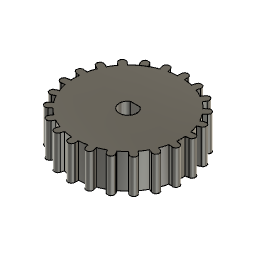
ZahnradProfilVorlage v5 (Autodesk Fusion 360 design; units mm, degrees)
Autodesk Fusion 360 part; units mm, degrees
note: some values were not read from the file. Chosen so that the rebuilt part matches the saved one: which face or edge a step refers to. Set by a fixed rule: which sketch regions a step uses.
sketch "Skizze1" plane through (0, 0, 0) normal (0, 0, 1) x (1, 0, 0)
  circle A0 centre (0, 0) radius 15.5076
  circle A1 centre (0, 16.5076) radius 1
  line L0 (-1, 16.5076) -> (1, 16.5076)
  line L1 (1, 16.5076) -> (1, 15.4753)
  line L2 (1, 15.4753) -> (-1, 15.4753)
  line L3 (-1, 15.4753) -> (-1, 16.5076)
  circle A2 centre (0, 0) radius 2.55
  line L4 (-1.4429, 2.1025) -> (1.4502, 2.0975)
  circle A3 centre (0, 0) radius 17.5076
  line L5 (-3.6912, 16.1206) -> (-3.4004, 15.1302)
  line L6 (-3.4004, 15.1302) -> (-5.3194, 14.5667)
  line L7 (-5.6102, 15.5572) -> (-3.6912, 16.1206)
  circle A4 centre (-4.6507, 15.8389) radius 1
  line L8 (-5.3194, 14.5667) -> (-5.6102, 15.5572)
  line L9 (-8.0834, 14.4277) -> (-7.5253, 13.5593)
  line L10 (-7.5253, 13.5593) -> (-9.2078, 12.478)
  line L11 (-9.7659, 13.3464) -> (-8.0834, 14.4277)
  circle A5 centre (-8.9247, 13.887) radius 1
  line L12 (-9.2078, 12.478) -> (-9.7659, 13.3464)
  line L13 (-11.8207, 11.5659) -> (-11.0406, 10.8899)
  line L14 (-11.0406, 10.8899) -> (-12.3503, 9.3784)
  line L15 (-13.1304, 10.0544) -> (-11.8207, 11.5659)
  circle A6 centre (-12.4756, 10.8102) radius 1
  line L16 (-12.3503, 9.3784) -> (-13.1304, 10.0544)
  line L17 (-14.6004, 7.7671) -> (-13.6614, 7.3383)
  line L18 (-13.6614, 7.3383) -> (-14.4922, 5.519)
  line L19 (-15.4312, 5.9479) -> (-14.6004, 7.7671)
  circle A7 centre (-15.0158, 6.8575) radius 1
  line L20 (-14.4922, 5.519) -> (-15.4312, 5.9479)
  line L21 (-16.1972, 3.3391) -> (-15.1755, 3.1922)
  line L22 (-15.1755, 3.1922) -> (-15.4601, 1.2125)
  line L23 (-16.4819, 1.3594) -> (-16.1972, 3.3391)
  circle A8 centre (-16.3395, 2.3493) radius 1
  line L24 (-15.4601, 1.2125) -> (-16.4819, 1.3594)
  line L25 (-16.4819, -1.3594) -> (-15.4601, -1.2125)
  line L26 (-15.4601, -1.2125) -> (-15.1755, -3.1922)
  line L27 (-16.1972, -3.3391) -> (-16.4819, -1.3594)
  circle A9 centre (-16.3395, -2.3493) radius 1
  line L28 (-15.1755, -3.1922) -> (-16.1972, -3.3391)
  line L29 (-15.4312, -5.9479) -> (-14.4922, -5.519)
  line L30 (-14.4922, -5.519) -> (-13.6614, -7.3383)
  line L31 (-14.6004, -7.7671) -> (-15.4312, -5.9479)
  circle A10 centre (-15.0158, -6.8575) radius 1
  line L32 (-13.6614, -7.3383) -> (-14.6004, -7.7671)
  line L33 (-13.1304, -10.0544) -> (-12.3503, -9.3784)
  line L34 (-12.3503, -9.3784) -> (-11.0406, -10.8899)
  line L35 (-11.8207, -11.5659) -> (-13.1304, -10.0544)
  circle A11 centre (-12.4756, -10.8102) radius 1
  line L36 (-11.0406, -10.8899) -> (-11.8207, -11.5659)
  line L37 (-9.7659, -13.3464) -> (-9.2078, -12.478)
  line L38 (-9.2078, -12.478) -> (-7.5253, -13.5593)
  line L39 (-8.0834, -14.4277) -> (-9.7659, -13.3464)
  circle A12 centre (-8.9247, -13.887) radius 1
  line L40 (-7.5253, -13.5593) -> (-8.0834, -14.4277)
  line L41 (-5.6102, -15.5572) -> (-5.3194, -14.5667)
  line L42 (-5.3194, -14.5667) -> (-3.4004, -15.1302)
  line L43 (-3.6912, -16.1206) -> (-5.6102, -15.5572)
  circle A13 centre (-4.6507, -15.8389) radius 1
  line L44 (-3.4004, -15.1302) -> (-3.6912, -16.1206)
  line L45 (-1, -16.5076) -> (-1, -15.4753)
  line L46 (-1, -15.4753) -> (1, -15.4753)
  line L47 (1, -16.5076) -> (-1, -16.5076)
  circle A14 centre (0, -16.5076) radius 1
  line L48 (1, -15.4753) -> (1, -16.5076)
  line L49 (3.6912, -16.1206) -> (3.4004, -15.1302)
  line L50 (3.4004, -15.1302) -> (5.3194, -14.5667)
  line L51 (5.6102, -15.5572) -> (3.6912, -16.1206)
  circle A15 centre (4.6507, -15.8389) radius 1
  line L52 (5.3194, -14.5667) -> (5.6102, -15.5572)
  line L53 (8.0834, -14.4277) -> (7.5253, -13.5593)
  line L54 (7.5253, -13.5593) -> (9.2078, -12.478)
  line L55 (9.7659, -13.3464) -> (8.0834, -14.4277)
  circle A16 centre (8.9247, -13.887) radius 1
  line L56 (9.2078, -12.478) -> (9.7659, -13.3464)
  line L57 (11.8207, -11.5659) -> (11.0406, -10.8899)
  line L58 (11.0406, -10.8899) -> (12.3503, -9.3784)
  line L59 (13.1304, -10.0544) -> (11.8207, -11.5659)
  circle A17 centre (12.4756, -10.8102) radius 1
  line L60 (12.3503, -9.3784) -> (13.1304, -10.0544)
  line L61 (14.6004, -7.7671) -> (13.6614, -7.3383)
  line L62 (13.6614, -7.3383) -> (14.4922, -5.519)
  line L63 (15.4312, -5.9479) -> (14.6004, -7.7671)
  circle A18 centre (15.0158, -6.8575) radius 1
  line L64 (14.4922, -5.519) -> (15.4312, -5.9479)
  line L65 (16.1972, -3.3391) -> (15.1755, -3.1922)
  line L66 (15.1755, -3.1922) -> (15.4601, -1.2125)
  line L67 (16.4819, -1.3594) -> (16.1972, -3.3391)
  circle A19 centre (16.3395, -2.3493) radius 1
  line L68 (15.4601, -1.2125) -> (16.4819, -1.3594)
  line L69 (16.4819, 1.3594) -> (15.4601, 1.2125)
  line L70 (15.4601, 1.2125) -> (15.1755, 3.1922)
  line L71 (16.1972, 3.3391) -> (16.4819, 1.3594)
  circle A20 centre (16.3395, 2.3493) radius 1
  line L72 (15.1755, 3.1922) -> (16.1972, 3.3391)
  line L73 (15.4312, 5.9479) -> (14.4922, 5.519)
  line L74 (14.4922, 5.519) -> (13.6614, 7.3383)
  line L75 (14.6004, 7.7671) -> (15.4312, 5.9479)
  circle A21 centre (15.0158, 6.8575) radius 1
  line L76 (13.6614, 7.3383) -> (14.6004, 7.7671)
  line L77 (13.1304, 10.0544) -> (12.3503, 9.3784)
  line L78 (12.3503, 9.3784) -> (11.0406, 10.8899)
  line L79 (11.8207, 11.5659) -> (13.1304, 10.0544)
  circle A22 centre (12.4756, 10.8102) radius 1
  line L80 (11.0406, 10.8899) -> (11.8207, 11.5659)
  line L81 (9.7659, 13.3464) -> (9.2078, 12.478)
  line L82 (9.2078, 12.478) -> (7.5253, 13.5593)
  line L83 (8.0834, 14.4277) -> (9.7659, 13.3464)
  circle A23 centre (8.9247, 13.887) radius 1
  line L84 (7.5253, 13.5593) -> (8.0834, 14.4277)
  line L85 (5.6102, 15.5572) -> (5.3194, 14.5667)
  line L86 (5.3194, 14.5667) -> (3.4004, 15.1302)
  line L87 (3.6912, 16.1206) -> (5.6102, 15.5572)
  circle A24 centre (4.6507, 15.8389) radius 1
  line L88 (3.4004, 15.1302) -> (3.6912, 16.1206)
  dimension "d2" = 2
  dimension "d13" = 5.1
  dimension "d24" = 35.0151
  dimension "d33" = 2.1
  dimension "d35" = 360
  constraint coincident A0.centre A2.centre
  constraint tangent A0 A1
  constraint perpendicular L0 L1
  constraint parallel L0 L2
  constraint parallel L1 L3
  constraint coincident A1 L0.end
  constraint horizontal L0
  constraint coincident A1 L0.start
  constraint coincident A0 L2.end
  constraint coincident A0 L1.end
  constraint coincident A2 L4.start
  constraint coincident A2 L4.end
  constraint concentric A0 A3
  constraint tangent A1 A3
  constraint tangent A1 L3
  measures "d2" diameter of A1
  measures "d13" diameter of A2
  measures "d24" diameter of A3
  measures "d33" distance of L4 A0.centre
extrude "Extrusion9" add sketch "Skizze1" along normal blind 10 contours A0 L2 L6 L10 L14 L18 L22 L26 L30 L34 L38 L42 L46 L50 L54 L58 L62 L66 L70 L74 L78 L82 L86 | A0 L70 | A0 L69 A20 | A0 A19 L68 | A0 L66 | A0 A20 L72 | L71 A20 | L71 A20 | A0 L65 A19 | L67 A19 | L67 A19 | A0 L74 | A0 L73 A21 | A0 A18 L64 | A0 L62 | A0 A21 L76 | L75 A21 | L75 A21 | A0 L61 A18 | L63 A18 | L63 A18 | A0 L78 | A0 L77 A22 | A0 A17 L60 | A0 L58 | L79 A22 | A0 A22 L80 | L79 A22 | L59 A17 | A0 L57 A17 | L59 A17 | L83 A23 | A0 L82 | A0 L81 A23 | L55 A16 | A0 A16 L56 | A0 L54 | L87 A24 | L83 A23 | A0 A23 L84 | L51 A15 | L55 A16 | A0 L53 A16 | A1 L0 | L87 A24 | A0 A24 L88 | A0 L86 | A0 L85 A24 | L47 A14 | L51 A15 | A0 L49 A15 | A0 A15 L52 | A0 L50 | A0 A1 L1 | A1 L0 | A0 A1 L3 | L7 A4 | L43 A13 | L47 A14 | A0 L45 A14 | A0 A14 L48 | A0 L2 | L11 A5 | L7 A4 | A0 L5 A4 | A0 A4 L8 | L39 A12 | L43 A13 | A0 L41 A13 | A0 A13 L44 | A0 L46 | A0 L6 | L15 A6 | L11 A5 | A0 L9 A5 | A0 A5 L12 | L35 A11 | L39 A12 | A0 L37 A12 | A0 A12 L40 | A0 L42 | L19 A7 | L15 A6 | A0 L13 A6 | A0 A6 L16 | L31 A10 | L35 A11 | A0 L33 A11 | A0 A11 L36 | A0 L38 | L23 A8 | L19 A7 | A0 L17 A7 | A0 A7 L20 | A0 L14 | L27 A9 | L31 A10 | A0 L29 A10 | A0 A10 L32 | A0 L34 | L23 A8 | A0 L21 A8 | A0 A8 L24 | A0 L18 | L27 A9 | A0 L25 A9 | A0 A9 L28 | A0 L30 | A0 L22 | A0 L26 | A2 L4 picked at (-0.3806, 2.1588)
equation "d24 = ( 22 * 5 ) / 3.1415 * 1 mm"
